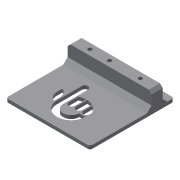
# Autodesk Inventor part: misc_hand_stand2
Saved by Autodesk Inventor 2014 (Build 180170000, 170)
## iProperties
Created: 2015-08-17
Part Number: misc_hand_stand2
Material: Generic
Document SubType Name: Modeling
Designer: Martin
Density: 1 g/cm^3
Appearance: Default
Author: Martin
Autodesk Inventor part; units mm, degrees
ref_plane "YZ Plane" through (0, 0, 0) normal (1, 0, 0) x (0, 1, 0)
ref_plane "XZ Plane" through (0, 0, 0) normal (0, 1, 0) x (-1, 0, 0)
ref_plane "XY Plane" through (0, 0, 0) normal (0, 0, 1) x (1, 0, 0)
sketch "Sketch1" plane through (0, 0, 0) normal (0, 0, 1) x (1, 0, 0)
  line L0 (-52.5, 0) -> (52.5, 0) projected
  line L1 (0, -52.5) -> (0, 52.5) projected
  line L2 (-37.5, -37.5) -> (37.5, -37.5)
  line L3 (37.5, -37.5) -> (37.5, 37.5)
  line L4 (37.5, 37.5) -> (-37.5, 37.5)
  line L5 (-37.5, 37.5) -> (-37.5, -37.5)
  line L6 (-37.5, -37.5) -> (37.5, 37.5) construction
  line L7 (37.5, -37.5) -> (-37.5, 37.5) construction
  point P0 (0, 0)
  dimension "d0" = 75
  dimension "d1" = 75
  constraints: 12 end point, 2 midpoint, 2 parallel, 1 horizontal, 1 perpendicular
  measures "d0" distance of L3.end L4.end
  measures "d1" distance of L2.end L3.end
extrude "Extrusion1" add sketch "Sketch1" along normal blind 3
sketch "Sketch2" plane through (0, 0, 3) normal (0, 0, 1) x (1, 0, 0)
  line L0 (37.5, -37.5) -> (37.5, 37.5) projected
  line L1 (37.5, 37.5) -> (-37.5, 37.5) projected
  line L2 (37.5, 17.5) -> (37.5, 27.5)
  line L3 (37.5, 27.5) -> (-37.5, 27.5)
  line L4 (-37.5, 27.5) -> (-37.5, 17.5)
  line L5 (-37.5, 17.5) -> (37.5, 17.5)
  point P0 (0, 0)
  dimension "d4" = 10
  dimension "d5" = 10
  constraints: 8 end point, 2 parallel, 2 point on line, 1 perpendicular
  measures "d4" distance between parallel lines of L1 L3
  measures "d5" distance between parallel lines of L5 L3
extrude "Extrusion2" add sketch "Sketch2" along normal blind 15
chamfer "Chamfer1" distance 2.5 angle 45 2 edges at (37.5, 22.5, 18) (-37.5, 22.5, 18)
sketch "Sketch3" plane through (0, 0, 18) normal (0, 0, 1) x (1, 0, 0)
  line L0 (-35, 17.5) -> (-35, 27.5) projected
  line L1 (35, 27.5) -> (35, 17.5) projected
  line L2 (-35, 22.5) -> (35, 22.5) construction
  circle A0 centre (-5, 22.5) radius 1.75
  circle A1 centre (-22.5, 22.5) radius 1.75
  line L3 (0, -52.5) -> (0, 52.5) projected
  circle A2 centre (22.5, 22.5) radius 1.75
  point P0 (0, 0)
  dimension "d11" = 45
  dimension "d12" = 17.5
  dimension "d13" = 5
  dimension "d14" = 3.5
  constraints: 3 centre point, 3 point on line, 2 end point, 2 equal radius, 2 midpoint
  measures "d11" distance of A2.centre A1.centre
  measures "d12" distance of A0.centre A1.centre
  measures "d13" distance from line of L3 A0.centre
  measures "d14" diameter of A2
extrude "Extrusion3" cut sketch "Sketch3" against normal through all
sketch "Sketch4" plane through (0, 0, 0) normal (0, 0, -1) x (-1, 0, 0)
  circle A0 centre (22.5, 22.5) radius 1.75 projected
  circle A1 centre (5, 22.5) radius 1.75 projected
  circle A2 centre (-22.5, 22.5) radius 1.75 projected
  circle A3 centre (-22.5, 22.5) radius 3.25
  circle A4 centre (5, 22.5) radius 3.25
  circle A5 centre (22.5, 22.5) radius 3.25
  point P0 (0, 0)
  dimension "d17" = 6.5
  constraints: 3 centre point, 3 coincident, 2 equal radius
  measures "d17" diameter of A5
extrude "Extrusion4" cut sketch "Sketch4" against normal blind 4
fillet "Fillet1" radius 2 4 edges at (37.5, -37.5, 1.5) (37.5, 37.5, 1.5) (-37.5, 37.5, 1.5) (-37.5, -37.5, 1.5)
sketch "Sketch5" plane through (0, 0, 3) normal (0, 0, 1) x (1, 0, 0)
  line L0 (0, -52.9971) -> (0, 52.5828) projected
  line L1 (7.5616, -15.7589) -> (7.5616, -16.8195) construction
  line L2 (7.1591, -15.7589) -> (12.7273, -15.7589)
  arc A0 (7.1591, -12.9748) -> (12.7273, -12.9748) centre (9.9432, -12.9748) ccw
  line L3 (0, -16.8195) -> (12.7273, -16.8195) construction
  arc A1 (0.5303, -12.9748) -> (6.0985, -12.9748) centre (3.3144, -12.9748) ccw
  line L4 (0, -29.5467) -> (12.7273, -29.5467) construction
  arc A2 (-7.1591, -16.8195) -> (7.1591, -16.8195) centre (0, -16.8195) ccw
  circle A3 centre (0, -16.8195) radius 7.1591 construction
  line L5 (0, -12.75) -> (0, 20.5)
  arc A4 (-12.7273, -16.8195) -> (12.7273, -16.8195) centre (0, -16.8195) ccw
  circle A5 centre (0, -16.8195) radius 12.7273 construction
  line L6 (7.1591, -16.8195) -> (12.7273, -16.8195)
  line L7 (-12.7273, -16.8195) -> (-12.7273, 5.4533)
  line L8 (-7.1591, -16.8195) -> (-7.1591, 5.4533)
  arc A6 (-7.1591, 5.4533) -> (-12.7273, 5.4533) centre (-9.9432, 5.4533) ccw
  line L9 (-6.0985, -9.3431) -> (-7.1591, -9.3431) construction
  line L10 (0.5303, -9.3431) -> (-0.5303, -9.3431) construction
  arc A7 (-0.5303, -4.1032) -> (-6.0985, -5.6484) centre (0, -16.8195) ccw
  arc A8 (-0.5303, -2.9376) -> (-6.0985, -4.3376) centre (0, -16.8195) ccw
  line L11 (6.0985, -2.9274) -> (6.0985, -15.7589)
  line L12 (7.1591, -2.9274) -> (7.1591, -15.7589)
  line L13 (12.7273, -15.7589) -> (12.7273, -2.9274)
  line L14 (12.7273, -2.9274) -> (7.1591, -2.9274)
  arc A9 (12.7273, -11.2513) -> (7.1591, -4.9142) centre (0, -16.8195) ccw
  line L15 (7.1591, -9.3431) -> (6.0985, -9.3431) construction
  line L16 (0.5303, -2.9274) -> (6.0985, -2.9274)
  line L17 (6.0985, -15.7589) -> (0.5303, -15.7589)
  arc A10 (6.0985, -5.6484) -> (0.5303, -4.1032) centre (0, -16.8195) ccw
  arc A11 (6.0985, -4.3376) -> (0.5303, -2.9376) centre (0, -16.8195) ccw
  arc A12 (12.7273, -11.2513) -> (-7.1591, -4.9142) centre (0, -16.8195) ccw construction
  line L18 (12.7273, -2.9274) -> (-7.1591, -2.9274) construction
  line L19 (0.5303, -15.7589) -> (0.5303, -2.9274)
  line L20 (-6.0985, -2.9274) -> (-0.5303, -2.9274)
  line L21 (-0.5303, -15.7589) -> (-6.0985, -15.7589)
  line L22 (-6.0985, -15.7589) -> (-6.0985, -2.9274)
  line L23 (-0.5303, -2.9274) -> (-0.5303, -15.7589)
  line L24 (-27.7979, -16.8195) -> (15.0178, -16.8195)
  line L25 (-6.0172, -28.1735) -> (-24.2274, -21.5455) construction
  line L26 (-13.7879, -7.274) -> (-12.7273, -7.274) construction
  line L27 (-13.7879, -7.274) -> (-19.3561, -5.2474) construction
  line L28 (-13.7879, -18.4104) -> (-13.7879, -7.274) construction
  line L29 (-13.7879, -18.4104) -> (-13.7879, -13.1995)
  line L30 (-19.3561, -10.4582) -> (-19.3561, -5.2474)
  arc A13 (-13.7879, -13.1995) -> (-19.3561, -5.2474) centre (-22.2504, -13.1995) ccw
  line L31 (-19.3561, -5.2474) -> (-19.3561, -16.3837) construction
  line L32 (-19.3561, -16.3837) -> (-13.7879, -18.4104) construction
  arc A14 (-19.3561, -10.4582) -> (-13.7879, -18.4104) centre (-10.8935, -10.4582) ccw
  arc A15 (-6.0985, -12.9748) -> (-0.5303, -12.9748) centre (-3.3144, -12.9748) ccw
  point P0 (0, 0)
  point P1 (0, 0)
  point P2 (12.683, -15.7589)
  point P3 (7.1591, -6.2966)
  dimension "d21" = 14.3182
  dimension "d22" = 5.5682
  dimension "d23" = 22.2727
  dimension "d24" = 0
  dimension "d25" = 5.5682
  dimension "d26" = 11.1364
  dimension "d27" = 1.5909
  dimension "d28" = 160
  dimension "d29" = 5.5682
  dimension "d30" = 1.0606
  dimension "d31" = 5.5682
  dimension "d32" = 32.0833
  dimension "d33" = 35
  constraints: 64 end point, 34 point on line, 33 point on circle, 20 tangent, 15 centre point, 11 parallel, 8 perpendicular, 6 equal length, 5 midpoint, 4 collinear, 4 concentric, 3 horizontal, 2 coincident, 2 vertical, 15 other
  measures "d21" diameter of A3
  measures "d23" distance from line of L24 A6.centre
  measures "d24" distance between parallel lines of L24 L3
  measures "d25" horizontal distance of L29.start L32.start
  measures "d26" distance of L32.start L27.end
  measures "d27" distance from line of L24 L29.start
  measures "d28" angle of L24 L25
  measures "d29" distance between parallel lines of L23 L22
  measures "d30" distance between parallel lines of L8 L22
  measures "d31" distance from line of L24 A12.start
  measures "d32" distance from line of L3.end L30
  measures "d33" distance from line of L4 A6.centre
extrude "ext_cut_logo" cut sketch "Sketch5" against normal through all contours A4 L24 A2 L0 | L29 A14 L24 | L24 A14 L30 A13 L29 | L0 A2 L6 A4 | L7 A6 L8 L24 | A0 L12 A9 L13 | L19 A10 L11 A1 | L19 A11 L11 A10 | L23 A15 L22 A7 | A7 L22 A8 L23
sketch "Sketch6" plane through (0, 0, 0) normal (0, 0, -1) x (-1, 0, 0)
  circle A0 centre (22.5, 22.5) radius 3.25 projected
  circle A1 centre (-22.5, 22.5) radius 3.25 projected
  circle A2 centre (5, 22.5) radius 3.25 projected
  circle A3 centre (-22.5, 22.5) radius 2.5
  circle A4 centre (5, 22.5) radius 2.5
  circle A5 centre (22.5, 22.5) radius 2.5
  point P0 (0, 0)
  dimension "d36" = 5
  constraints: 3 centre point, 3 coincident, 2 equal radius
  measures "d36" diameter of A3
extrude "PRINT_support" add sketch "Sketch6" against normal blind 3.5 contours A3 | A4 | A5
chamfer "Chamfer2" distance 4 angle 45 2 edges at (0, 17.5, 3) (0, 27.5, 3)
equation "\"d21\" = 0.409091 * d33"
equation "\"d22\" = d31"
equation "\"d23\" = 0.636364 * d33"
equation "\"d25\" = d31"
equation "\"d26\" = 0.318182 * d33"
equation "\"d27\" = 0.0454545 * d33"
equation "\"d29\" = d31"
body "Solid1"
